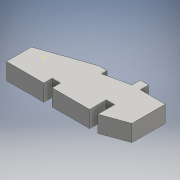
# Autodesk Inventor part: 240405_sketch2
Saved by Autodesk Inventor 2016 (Build 200138000, 138)
## iProperties
Created: 2024-04-05
Part Number: 240405_sketch2
Material: 일반
Document SubType Name: Modeling
Designer: pc
Density: 1 g/cm^3
Appearance: 기본값
Author: pc
Autodesk Inventor part; units mm, degrees
ref_plane "YZ Plane" through (0, 0, 0) normal (1, 0, 0) x (0, 1, 0)
ref_plane "XZ Plane" through (0, 0, 0) normal (0, 1, 0) x (-1, 0, 0)
ref_plane "XY Plane" through (0, 0, 0) normal (0, 0, 1) x (1, 0, 0)
sketch "스케치1" plane through (0, 0, 0) normal (0, 0, 1) x (1, 0, 0)
  line L0 (-17.9543, 3.9382) -> (-17.9543, -26.0618)
  line L1 (-17.9543, -26.0618) -> (27.0457, -26.0618)
  line L2 (27.0457, -26.0618) -> (27.0457, -16.0618)
  line L3 (27.0457, -16.0618) -> (37.0457, -16.0618)
  line L4 (37.0457, -16.0618) -> (37.0457, -26.0618)
  line L5 (37.0457, -26.0618) -> (82.0457, -26.0618)
  line L6 (82.0457, -26.0618) -> (82.0457, -6.0618)
  line L7 (82.0457, -6.0618) -> (92.0457, -6.0618)
  line L8 (92.0457, -6.0618) -> (92.0457, -26.0618)
  line L9 (92.0457, -26.0618) -> (122.0457, -15.1427)
  line L10 (122.0457, -15.1427) -> (122.0457, 24.8573)
  line L11 (122.0457, 24.8573) -> (92.0457, 24.8573)
  line L12 (92.0457, 24.8573) -> (92.0457, 34.8573)
  line L13 (92.0457, 34.8573) -> (82.0457, 34.8573)
  line L14 (82.0457, 34.8573) -> (82.0457, 24.8573)
  line L15 (82.0457, 24.8573) -> (52.0457, 18.1338)
  line L16 (52.0457, 18.1338) -> (52.0457, 24.8573)
  line L17 (52.0457, 24.8573) -> (42.0457, 24.8573)
  line L18 (42.0457, 24.8573) -> (-17.9543, 3.9382)
  point P0 (0, 0)
  dimension "d0" = 30
  dimension "d1" = 45
  dimension "d2" = 10
  dimension "d3" = 10
  dimension "d4" = 45
  dimension "d5" = 20
  dimension "d6" = 10
  dimension "d8" = 20
  dimension "d9" = 30
  dimension "d10" = 40
  dimension "d11" = 30
  dimension "d12" = 10
  dimension "d13" = 10
  dimension "d14" = 30
  dimension "d15" = 10
  dimension "d16" = 140
  constraints: 38 end point, 11 perpendicular, 4 point on line, 3 vertical, 1 horizontal
  measures "d0" distance of L0.start L0.end
  measures "d1" distance of L0.end L1.end
  measures "d2" distance of L1.end L2.end
  measures "d3" distance of L2.end L3.end
  measures "d4" distance of L4.end L5.end
  measures "d5" distance of L5.end L6.end
  measures "d6" distance of L6.end L7.end
  measures "d8" angle of L5 L9
  measures "d9" distance from line of L9.end L8
  measures "d10" distance of L9.end L10.end
  measures "d11" distance of L10.end L11.end
  measures "d12" distance of L11.end L12.end
  measures "d13" distance of L12.end L13.end
  measures "d14" horizontal distance of L15.end L14.end
  measures "d15" distance of L16.end L17.end
  measures "d16" distance between parallel lines of L10 L0
extrude "돌출1" add sketch "스케치1" along normal blind 20
sketch "스케치2" plane through (0, 0, 20) normal (0, 0, 1) x (1, 0, 0)
  point P0 (0, 0)
